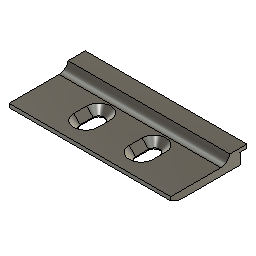
Microfluidic Clamp (Autodesk Fusion 360 design; units mm, degrees)
Autodesk Fusion 360 part; units mm, degrees
sketch "Sketch1" plane through (0, 0, 0) normal (0, 0, 1) x (1, 0, 0)
  line L0 (17.5, -7.5) -> (-17.5, -7.5)
  line L1 (-17.5, -7.5) -> (-17.5, 7.5)
  line L2 (-17.5, 7.5) -> (17.5, 7.5)
  line L3 (17.5, 7.5) -> (17.5, -7.5)
  line L4 (17.5, -7.5) -> (-17.5, 7.5) construction
  line L5 (-17.5, -7.5) -> (17.5, 7.5) construction
  dimension "d1" = 35
  dimension "d2" = 15
  constraint perpendicular L0 L1
  constraint parallel L0 L2
  constraint parallel L1 L3
  constraint horizontal L0
  constraint coincident L4 origin
  constraint coincident L5 origin
  measures "d1" distance of L1.end L2.end
  measures "d2" distance of L0.start L2.end
extrude "Extrude1" add sketch "Sketch1" along normal blind 1.6
sketch "Sketch2" plane through (17.5, 0, 0) normal (1, 0, 0) x (0, 1, 0)
  line L0 (-7.5, 0) -> (7.5, 0)
  line L1 (7.5, 0) -> (7.5, 1.6)
  line L2 (7.5, 1.6) -> (-7.5, 1.6)
  line L3 (-7.5, 1.6) -> (-7.5, 0)
  line L4 (-5.5, 0) -> (-7.5, 0.8)
  line L5 (-7.5, 0.8) -> (-7.5, 0)
  line L6 (-7.5, 0) -> (-5.5, 0)
  dimension "d5" = 2
  constraint coincident L0 L4.start
  constraint midpoint L3 L4.end
  constraint coincident L0.start L3.end
  measures "d5" distance of L4.start L0.start
extrude "Extrude2" cut sketch "Sketch2" against normal up to surface (35 mm away) contours L0 L3 L4 L5 L6
sketch "Sketch3" plane through (0, 0, 1.6) normal (0, 0, 1) x (-1, 0, 0)
  line L0 (-17.5, -7.5) -> (17.5, -7.5)
  line L1 (17.5, -7.5) -> (17.5, 7.5)
  line L2 (17.5, 7.5) -> (-17.5, 7.5)
  line L3 (-17.5, 7.5) -> (-17.5, -7.5)
  line L4 (17.5, -7.5) -> (-17.5, -7.5)
  line L5 (-17.5, -7.5) -> (-17.5, -5.3)
  line L6 (-17.5, -5.3) -> (17.5, -5.3)
  line L7 (17.5, -5.3) -> (17.5, -7.5)
  dimension "d8" = 2.2
  constraint horizontal L4
  constraint vertical L5
  constraint horizontal L6
  constraint vertical L7
  constraint coincident L3 L5.end
  constraint coincident L0.end L1.start
  measures "d8" distance of L0.start L5.end
extrude "Extrude3" add sketch "Sketch3" along normal blind 1.6 contours L0 L1 L3 L4 L5 L6 L7
fillet "Fillet1" radius 2 1 edges at (0, 5.3, 1.6)
sketch "Sketch4" plane through (0, 7.5, 0) normal (0, 1, 0) x (-1, 0, 0)
  line L0 (-17.5, 0) -> (17.5, 0)
  line L1 (17.5, 0) -> (17.5, 3.2)
  line L2 (17.5, 3.2) -> (-17.5, 3.2)
  line L3 (-17.5, 3.2) -> (-17.5, 0)
  line L4 (-17.5, 3.2) -> (17.5, 3.2)
  line L5 (17.5, 3.2) -> (17.5, 2.4)
  line L6 (17.5, 2.4) -> (-17.5, 2.4)
  line L7 (-17.5, 2.4) -> (-17.5, 3.2)
  line L8 (17.5, 1.6) -> (17.5, 3.2)
  dimension "d12" = 1
  constraint horizontal L4
  constraint vertical L5
  constraint horizontal L6
  constraint vertical L7
  constraint midpoint L5.end L8
  constraint coincident L2.end L3.start
extrude "Extrude4" add sketch "Sketch4" along normal blind 1.5 contours L1 L2 L3 L4 L5 L6 L7 L8
sketch "Sketch5" plane through (0, 0, 1.6) normal (0, 0, 1) x (-1, 0, 0)
  line L0 (-17.5, -3.3404) -> (17.5, -3.3404)
  line L1 (17.5, -3.3404) -> (17.5, 7.5)
  line L2 (17.5, 7.5) -> (-17.5, 7.5)
  line L3 (-17.5, 7.5) -> (-17.5, -3.3404)
  line L4 (6, 1) -> (-6, 1)
  line L5 (4.8, 2.4) -> (7.2, 2.4)
  line L6 (7.2, 2.4) -> (7.2, -0.4)
  line L7 (7.2, -0.4) -> (4.8, -0.4)
  line L8 (4.8, -0.4) -> (4.8, 2.4)
  line L9 (4.8, 2.4) -> (7.2, -0.4) construction
  line L10 (7.2, 2.4) -> (4.8, -0.4) construction
  arc A0 (4.8, -0.4) -> (7.2, -0.4) centre (6, -0.4) ccw
  arc A1 (7.2, 2.4) -> (4.8, 2.4) centre (6, 2.4) ccw
  line L11 (0, -1.5) -> (0, 7.5)
  arc A2 (-4.8, 2.4) -> (-7.2, 2.4) centre (-6, 2.4) ccw
  arc A3 (-7.2, -0.4) -> (-4.8, -0.4) centre (-6, -0.4) ccw
  line L12 (-4.8, 2.4) -> (-7.2, 2.4)
  line L13 (-4.8, 2.4) -> (-7.2, -0.4) construction
  line L14 (-4.8, -0.4) -> (-4.8, 2.4)
  line L15 (-7.2, 2.4) -> (-7.2, -0.4)
  line L16 (-7.2, 2.4) -> (-4.8, -0.4) construction
  line L17 (-7.2, -0.4) -> (-4.8, -0.4)
  line L18 (17.5, -7.5) -> (-17.5, -7.5)
  point P0 (0, 1)
  point P1 (6, 1)
  point P2 (-6, 1)
  point P3 (-6, 1)
  dimension "d15" = 12
  dimension "d18" = 2.4
  dimension "d19" = 2.8
  dimension "d20" = 1.2
  dimension "d21" = 1.2
  dimension "d25" = 8.5
  constraint parallel L0 L4
  constraint midpoint L4 P0
  constraint vertical origin P0
  constraint perpendicular L5 L6
  constraint parallel L5 L7
  constraint parallel L6 L8
  constraint horizontal L5
  constraint coincident L9 P1
  constraint coincident L10 P1
  constraint coincident P1 L4.start
  constraint midpoint L7 A0.centre
  constraint midpoint L5 A1.centre
  constraint midpoint L2 L11.end
  constraint perpendicular L2 L11
  constraint symmetric P1 L11 P3
  constraint symmetric L5.start L11 A2.start
  constraint symmetric L5.end L11 A2.end
  constraint symmetric L6.end L11 A3.start
  constraint symmetric L7.end L11 A3.end
  constraint symmetric A0 L11 A3
  constraint symmetric A1 L11 A2
  measures "d15" distance of P1 P3
  measures "d18" distance of L5.start L5.end
  measures "d19" distance of L5.end L6.end
  measures "d20" radius of A0
  measures "d21" radius of A1
  measures "d25" distance of L4 L18
extrude "Extrude5" cut sketch "Sketch5" against normal up to surface (1.6 mm away) contours L5 A1 | L5 L6 L7 L8 | L7 A0 | A2 L12 | L12 L14 L15 L17 | A3 L17
chamfer "Chamfer1" distance 1.4 angle 45 8 edges at (-6, -3.6, 1.6) (-7.2, -1, 1.6) (-6, 1.6, 1.6) (-4.8, -1, 1.6) (4.8, -1, 1.6) (6, 1.6, 1.6) (7.2, -1, 1.6) (6, -3.6, 1.6)
fillet "Fillet2" radius 1 1 edges at (0, -5.5, 0)
